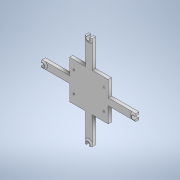
# Autodesk Inventor part: MiniCopterChassisV1
Saved by Autodesk Inventor 2020 (Build 240168000, 168)
## iProperties
Created: 2023-02-14
Part Number: MiniCopterChassisV1
Material: Generic
Document SubType Name: Modeling
Designer: agraa4529
Density: 1 g/cm^3
Appearance: Default
Author: agraa4529
Autodesk Inventor part; units mm, degrees
ref_plane "YZ Plane" through (0, 0, 0) normal (1, 0, 0) x (0, 1, 0)
ref_plane "XZ Plane" through (0, 0, 0) normal (0, 1, 0) x (-1, 0, 0)
ref_plane "XY Plane" through (0, 0, 0) normal (0, 0, 1) x (1, 0, 0)
sketch "Sketch1" plane through (0, 0, 0) normal (0, 0, 1) x (1, 0, 0)
  line L0 (-42, 42) -> (42, 42)
  line L1 (42, 42) -> (42, -42)
  line L2 (42, -42) -> (-42, -42)
  line L3 (-42, -42) -> (-42, 42)
  line L4 (-42, 42) -> (42, -42) construction
  line L5 (42, 42) -> (-42, -42) construction
  line L6 (-7.5, -18) -> (7.5, -18)
  line L7 (7.5, -18) -> (7.5, 102)
  line L8 (7.5, 102) -> (-7.5, 102)
  line L9 (-7.5, 102) -> (-7.5, -18)
  line L10 (-7.5, -18) -> (7.5, 102) construction
  line L11 (7.5, -18) -> (-7.5, 102) construction
  line L12 (-102, 7.5) -> (-102, -7.5)
  line L13 (18, 7.5) -> (-102, 7.5)
  line L14 (18, 7.5) -> (-102, -7.5) construction
  line L15 (-102, -7.5) -> (18, -7.5)
  line L16 (18, -7.5) -> (-102, 7.5) construction
  line L17 (18, -7.5) -> (18, 7.5)
  line L18 (-7.5, -102) -> (7.5, -102)
  line L19 (-7.5, 18) -> (-7.5, -102)
  line L20 (-7.5, 18) -> (7.5, -102) construction
  line L21 (7.5, -102) -> (7.5, 18)
  line L22 (7.5, 18) -> (-7.5, -102) construction
  line L23 (7.5, 18) -> (-7.5, 18)
  line L24 (102, -7.5) -> (102, 7.5)
  line L25 (-18, -7.5) -> (102, -7.5)
  line L26 (-18, -7.5) -> (102, 7.5) construction
  line L27 (102, 7.5) -> (-18, 7.5)
  line L28 (-18, 7.5) -> (102, -7.5) construction
  line L29 (-18, 7.5) -> (-18, -7.5)
  point P0 (0, 0)
  point P1 (0, 42)
  point P2 (-42, 0)
  point P3 (0, -42)
  point P4 (42, 0)
  point P5 (7.5, -42)
  point P6 (42, -7.5)
  point P7 (42, 7.5)
  point P8 (7.5, 42)
  point P9 (-7.5, 42)
  point P10 (-42, 7.5)
  point P11 (-42, -7.5)
  point P12 (-7.5, -42)
  dimension "d0" = 84
  dimension "d1" = 84
  dimension "d2" = 120
  dimension "d3" = 15
  dimension "d6" = 360
  constraints: 60 end point, 11 midpoint, 4 parallel, 2 horizontal, 2 perpendicular, 45 other
  measures "d0" distance of L0.start L0.end
  measures "d1" distance of L0.end L1.end
  measures "d2" distance of L6.end L7.end
  measures "d3" distance of L6.start L6.end
extrude "Extrusion1" add sketch "Sketch1" along normal blind 7
sketch "Sketch2" plane through (0, 0, 7) normal (0, 0, 1) x (1, 0, 0)
  line L0 (-32.85, 22.65) -> (32.85, 22.65)
  line L1 (32.85, 22.65) -> (32.85, -22.65)
  line L2 (32.85, -22.65) -> (-32.85, -22.65)
  line L3 (-32.85, -22.65) -> (-32.85, 22.65)
  line L4 (-32.85, 22.65) -> (32.85, -22.65) construction
  line L5 (32.85, 22.65) -> (-32.85, -22.65) construction
  circle A0 centre (-32.85, 22.65) radius 1.9
  circle A1 centre (32.85, 22.65) radius 1.9
  circle A2 centre (32.85, -22.65) radius 1.9
  circle A3 centre (-32.85, -22.65) radius 1.9
  point P0 (0, 0)
  dimension "d10" = 65.7
  dimension "d11" = 45.3
  dimension "d12" = 3.8
  dimension "d13" = 3.8
  dimension "d14" = 3.8
  dimension "d15" = 3.8
  constraints: 12 end point, 4 centre point, 4 coincident, 2 midpoint, 2 parallel, 1 horizontal, 1 perpendicular
  measures "d10" distance of L0.start L0.end
  measures "d11" distance of L2.end L0.start
  measures "d12" diameter of A0
  measures "d13" diameter of A1
  measures "d14" diameter of A2
  measures "d15" diameter of A3
extrude "Extrusion2" cut sketch "Sketch2" against normal blind 7 contours L3 A0 L0 | L0 A0 L3 | A1 L1 L0 | L0 L1 A1 | A3 L2 L3 | L3 L2 A3 | A2 L2 L1 | L1 L2 A2
sketch "Sketch3" plane through (0, 0, 0) normal (0, 0, -1) x (-1, 0, 0)
  circle A0 centre (32.85, 22.65) radius 1.9 projected
  circle A1 centre (32.85, 22.65) radius 3.5
  circle A2 centre (32.85, -22.65) radius 1.9 projected
  circle A3 centre (32.85, -22.65) radius 3.5
  circle A4 centre (-32.85, 22.65) radius 1.9 projected
  circle A5 centre (-32.85, 22.65) radius 3.5
  circle A6 centre (-32.85, -22.65) radius 3.5
  point P0 (0, 0)
  dimension "d18" = 7
  dimension "d19" = 7
  dimension "d20" = 7
  dimension "d21" = 7
  constraints: 4 centre point, 3 coincident
  measures "d18" diameter of A1
  measures "d19" diameter of A3
  measures "d20" diameter of A6
  measures "d21" diameter of A5
extrude "Extrusion3" cut sketch "Sketch3" against normal blind 4 contours A0 | A1 | A2 | A3 | A4 | A5 | A6
sketch "Sketch4" plane through (0, 0, 7) normal (0, 0, 1) x (1, 0, 0)
  line L0 (-102, 7.5) -> (-102, -7.5) projected
  line L1 (-102, 0) -> (-102, -3.16)
  line L2 (-102, 0) -> (-102, 3.16)
  line L3 (-102, 0) -> (-99.35, 0)
  circle A0 centre (-99.35, 0) radius 4.1241
  circle A1 centre (0, -99.35) radius 4.1241
  circle A2 centre (99.35, 0) radius 4.1241
  circle A3 centre (0, 99.35) radius 4.1241
  point P0 (0, 0)
  point P1 (-3.16, -102)
  point P2 (102, -3.16)
  point P3 (3.16, 102)
  dimension "d24" = 3.16
  dimension "d25" = 3.16
  dimension "d26" = 2.65
  dimension "d29" = 360
  constraints: 6 end point, 2 point on line, 1 coincident, 1 midpoint, 1 perpendicular, 25 other
  measures "d24" distance of L1.start L1.end
  measures "d25" distance of L1.start L2.end
  measures "d26" distance of L1.start L3.end
extrude "Extrusion4" cut sketch "Sketch4" against normal blind 7
sketch "Sketch5" plane through (0, 0, 7) normal (0, 0, 1) x (1, 0, 0)
  line L0 (-102, 7.5) -> (-102, 3.16) projected
  line L1 (-102, 3.16) -> (-96.7, -3.16)
  arc A0 (-102, -3.16) -> (-102, 3.16) centre (-99.35, 0) ccw projected
  arc A1 (-102, -4.6648) -> (-102, 4.6648) centre (-99.35, 0) ccw
  arc A2 (-102, -3.16) -> (-102, 3.16) centre (-99.35, 0) ccw
  line L2 (-102, 3.16) -> (-102, 4.6648)
  line L3 (-102, -3.16) -> (-102, -4.6648)
  line L4 (-102, -3.16) -> (-102, -7.5) projected
  arc A3 (4.6648, -102) -> (-4.6648, -102) centre (0, -99.35) ccw
  arc A4 (3.16, -102) -> (-3.16, -102) centre (0, -99.35) ccw
  line L5 (-3.16, -102) -> (-4.6648, -102)
  line L6 (3.16, -102) -> (4.6648, -102)
  arc A5 (102, 4.6648) -> (102, -4.6648) centre (99.35, 0) ccw
  arc A6 (102, 3.16) -> (102, -3.16) centre (99.35, 0) ccw
  line L7 (102, -3.16) -> (102, -4.6648)
  line L8 (102, 3.16) -> (102, 4.6648)
  arc A7 (-4.6648, 102) -> (4.6648, 102) centre (0, 99.35) ccw
  arc A8 (-3.16, 102) -> (3.16, 102) centre (0, 99.35) ccw
  line L9 (3.16, 102) -> (4.6648, 102)
  line L10 (-3.16, 102) -> (-4.6648, 102)
  point P0 (0, 0)
  dimension "d33" = 10.73
  dimension "d36" = 360
  constraints: 19 end point, 17 point on circle, 8 centre point, 5 coincident, 2 point on line, 1 concentric, 41 other
  measures "d33" diameter of A1
extrude "Extrusion5" add sketch "Sketch5" along normal blind 2.5 contours A1 L3 A0 L0 | L6 A4 L5 A3 | L8 A6 L7 A5 | L10 A8 L9 A7
fillet "Fillet1" radius 4 4 edges at (0, 93.985, 7) (93.985, 0, 7) (0, -93.985, 7) (-93.985, 0, 7)
body "Solid1"
